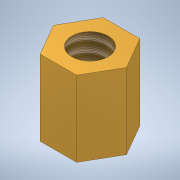
# Autodesk Inventor part: 22_Hexnut_5mm
Saved by Autodesk Inventor 2022.2 (Build 262287010, 287A)
## iProperties
Created: 2022-05-02
Part Number: 22_Hexnut_5mm
Material: Messing, weicher Gelbton
Document SubType Name: Modeling
Designer: MXBD
Density: 8.47 g/cm^3
Appearance: Messing - satiniert
Author: MXBD
Autodesk Inventor part; units mm, degrees
ref_plane "YZ Plane" through (0, 0, 0) normal (1, 0, 0) x (0, 1, 0)
ref_plane "XZ Plane" through (0, 0, 0) normal (0, 1, 0) x (-1, 0, 0)
ref_plane "XY Plane" through (0, 0, 0) normal (0, 0, 1) x (1, 0, 0)
sketch "Skizze1" plane through (0, 0, 0) normal (0, 1, 0) x (-1, 0, 0)
  line L0 (2.6558, 0) -> (1.3279, -2.3)
  line L1 (1.3279, -2.3) -> (-1.3279, -2.3)
  line L2 (-1.3279, -2.3) -> (-2.6558, 0)
  line L3 (-2.6558, 0) -> (-1.3279, 2.3)
  line L4 (-1.3279, 2.3) -> (1.3279, 2.3)
  line L5 (1.3279, 2.3) -> (2.6558, 0)
  line L6 (0, -3.22) -> (0, 3.22) projected
  line L7 (-3.7181, 0) -> (3.7181, 0) projected
  point P0 (0, 0)
  point P1 (0, 0)
  dimension "d0" = 4.6
  constraints: 12 end point, 1 coincident, 1 point on line, 13 other
  measures "d0" distance between parallel lines of L1 L4
extrude "Extrusion1" add sketch "Skizze1" along normal mid plane 5.5
sketch "Skizze2" plane through (0, 2.75, 0) normal (0, 1, 0) x (1, 0, 0)
  point P0 (0, 0)
  point P1 (0, 0)
  constraints: 1 coincident
hole "Bohrung1" at (0, 2.75, 0) direction (0, -1, 0) diameter 2.6416 end through all thread size "6-32 UNC" class "2B" standard "ANSI Unified Screw Threads"
